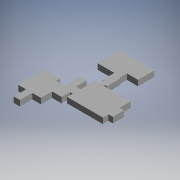
# Autodesk Inventor part: floormap2
Saved by Autodesk Inventor 2019.4 (Build 234330000, 330)
## iProperties
Part Number: floormap2
Material: Generic
Document SubType Name: Modeling
Designer: Jorge
Appearance: Default
Author: Jorge
Autodesk Inventor part; units mm, degrees
ref_plane "YZ Plane" through (0, 0, 0) normal (1, 0, 0) x (0, 1, 0)
ref_plane "XZ Plane" through (0, 0, 0) normal (0, 1, 0) x (-1, 0, 0)
ref_plane "XY Plane" through (0, 0, 0) normal (0, 0, 1) x (1, 0, 0)
sketch "Sketch1" plane through (0, 0, 0) normal (0, 1, 0) x (-1, 0, 0)
  line L0 (0, 0) -> (0, -2000)
  line L1 (0, 0) -> (800, 0)
  line L2 (800, 0) -> (800, 1000)
  line L3 (800, 1000) -> (7200, 1000)
  line L4 (7200, 1000) -> (7200, 0)
  line L5 (7200, 0) -> (7200, -1400) construction
  line L6 (0, -2000) -> (800, -2000)
  line L7 (800, -2000) -> (800, -4000)
  line L8 (800, -4000) -> (7200, -4000) construction
  line L9 (7200, -1400) -> (7200, -4000)
  line L10 (7200, -4000) -> (6500, -4000)
  line L11 (6500, -4000) -> (5700, -4000) construction
  line L12 (5700, -4000) -> (800, -4000)
  line L13 (7200, 0) -> (7700, 0)
  line L14 (7700, 0) -> (7700, 1500)
  line L15 (7700, 1500) -> (9400, 1500)
  line L16 (9400, 1500) -> (9400, 3500)
  line L17 (9400, 3500) -> (10950, 3500)
  line L18 (10950, 3500) -> (12050, 3500) construction
  line L19 (7200, -1400) -> (8000, -1400)
  line L20 (8000, -1400) -> (8000, -3300)
  line L21 (8000, -3300) -> (9200, -3300)
  line L22 (9200, -3300) -> (9200, -500)
  line L23 (9200, -500) -> (10650, -500)
  line L24 (10650, -500) -> (10650, -1200)
  line L25 (10650, -1200) -> (13450, -1200)
  line L26 (13450, -1200) -> (13450, 3500)
  line L27 (13450, 3500) -> (12050, 3500)
  line L28 (12050, 3500) -> (12050, 5700)
  line L29 (12050, 5700) -> (10950, 5700)
  line L30 (10950, 5700) -> (10950, 3500)
  line L31 (6500, -4000) -> (6500, -4850)
  line L32 (6500, -4850) -> (6700, -4850)
  line L33 (6700, -4850) -> (6700, -6950)
  line L34 (6700, -6950) -> (9700, -6950)
  line L35 (9700, -6950) -> (9700, -10950)
  line L36 (5700, -4000) -> (5700, -4200)
  line L37 (5700, -4200) -> (5300, -4200)
  line L38 (5300, -4200) -> (5300, -6650)
  line L39 (5300, -6650) -> (5500, -6650)
  line L40 (5500, -6650) -> (5500, -8000)
  line L41 (5500, -8000) -> (3500, -8000)
  line L42 (9700, -10950) -> (3500, -10950)
  line L43 (3500, -10950) -> (3500, -8000)
  dimension "d0" = 2000
  dimension "d1" = 800
  dimension "d2" = 1000
  dimension "d3" = 6400
  dimension "d4" = 1000
  dimension "d5" = 1400
  dimension "d6" = 2000
  dimension "d7" = 700
  dimension "d8" = 800
  dimension "d9" = 500
  dimension "d10" = 1500
  dimension "d11" = 1700
  dimension "d12" = 2000
  dimension "d13" = 1550
  dimension "d14" = 1100
  dimension "d15" = 800
  dimension "d16" = 1900
  dimension "d17" = 1200
  dimension "d18" = 2800
  dimension "d19" = 1450
  dimension "d20" = 700
  dimension "d21" = 2800
  dimension "d22" = 2200
  dimension "d23" = 850
  dimension "d24" = 200
  dimension "d25" = 2100
  dimension "d26" = 3000
  dimension "d27" = 4000
  dimension "d28" = 200
  dimension "d29" = 400
  dimension "d30" = 2450
  dimension "d31" = 200
  dimension "d32" = 1350
  dimension "d33" = 2000
  constraints: 88 end point, 28 perpendicular, 6 horizontal, 5 point on line, 4 vertical, 2 collinear, 1 coincident
  measures "d0" distance of L0.start L0.end
  measures "d1" distance of L0.start L1.end
  measures "d2" distance of L1.end L2.end
  measures "d3" distance of L2.end L3.end
  measures "d4" distance of L3.end L4.end
  measures "d5" distance of L4.end L5.end
  measures "d6" distance of L6.end L7.end
  measures "d7" distance of L8.end L10.end
  measures "d8" distance of L10.end L11.end
  measures "d9" distance of L4.end L13.end
  measures "d10" distance of L13.end L14.end
  measures "d11" distance of L14.end L15.end
  measures "d12" distance of L15.end L16.end
  measures "d13" distance of L16.end L17.end
  measures "d14" distance of L17.end L18.end
  measures "d15" distance of L5.end L19.end
  measures "d16" distance of L19.end L20.end
  measures "d17" distance of L20.end L21.end
  measures "d18" distance of L21.end L22.end
  measures "d19" distance of L22.end L23.end
  measures "d20" distance of L23.end L24.end
  measures "d21" distance of L24.end L25.end
  measures "d22" distance of L18.end L28.end
  measures "d23" distance of L10.end L31.end
  measures "d24" distance of L31.end L32.end
  measures "d25" distance of L32.end L33.end
  measures "d26" distance of L33.end L34.end
  measures "d27" distance of L34.end L35.end
  measures "d28" distance of L11.end L36.end
  measures "d29" distance of L36.end L37.end
  measures "d30" distance of L37.end L38.end
  measures "d31" distance of L38.end L39.end
  measures "d32" distance of L39.end L40.end
  measures "d33" distance of L40.end L41.end
extrude "Extrusion1" add sketch "Sketch1" along normal blind 1000
body "Solid1"
